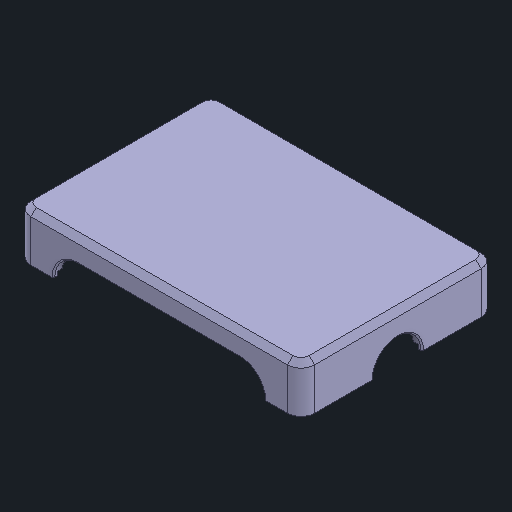
# Autodesk Inventor part: case2
Saved by Autodesk Inventor 2026.2 (Build 302298000, 298)
## iProperties
Created: 2025-10-05
Part Number: case2
Material: Generic
Document SubType Name: Modeling
Designer: micyg
Density: 1 g/cm^3
Appearance: Default
Sheet Metal Rule: Default
Author: micyg
## iProperties of the stored document case2_3DPrint.ipt
Created: 2025-10-05
Part Number: case2_3DPrint
Material: Generic
Document SubType Name: Modeling
Designer: micyg
Density: 1 g/cm^3
Appearance: Default
Author: micyg
Autodesk Inventor part; units mm, degrees
ref_plane "YZ Plane" through (0, 0, 0) normal (1, 0, 0) x (0, 1, 0)
ref_plane "XZ Plane" through (0, 0, 0) normal (0, 1, 0) x (-1, 0, 0)
ref_plane "XY Plane" through (0, 0, 0) normal (0, 0, 1) x (1, 0, 0)
sketch "Sketch1" plane through (0, 0, 0) normal (0, 1, 0) x (-1, 0, 0)
  line L0 (0, 0) -> (104.9, 0)
  line L1 (104.9, 0) -> (104.9, -71.6)
  line L2 (104.9, -71.6) -> (0, -71.6)
  line L3 (0, -71.6) -> (0, 0)
  dimension "d0" = 104.9
  dimension "d1" = 71.6
  constraints: 8 end point, 2 parallel, 1 horizontal, 1 perpendicular
  measures "d0" distance of L1.end L2.end
  measures "d1" distance of L0.end L1.end
extrude "Extrusion1" add sketch "Sketch1" along normal blind 17.5
fillet "Fillet1" radius 5 4 edges at (-104.9, 8.75, 0) (0, 8.75, 0) (-104.9, 8.75, -71.6) (0, 8.75, -71.6)
chamfer "Chamfer1" distance 2 angle 45 8 edges at (-52.45, 17.5, 0) (-1.4645, 17.5, -1.4645) (0, 17.5, -35.8) (-1.4645, 17.5, -70.1355) (-52.45, 17.5, -71.6) (-103.4355, 17.5, -70.1355) (-104.9, 17.5, -35.8) (-103.4355, 17.5, -1.4645)
shell "Shell2" thickness 3 removed faces 1 at (-68.2667, 0, -47.7333)
ref_plane "Work Plane2" through (-52.45, 0, 0) normal (1, 0, 0) x (0, 1, 0)
ref_plane "Work Plane3" through (0, 0, -35.8) normal (0, 0, -1) x (-1, 0, 0)
ref_plane "Work Plane4" through (0, 1.915, 0) normal (0, -1, 0) x (1, 0, 0)
sketch "Sketch19" plane through (-52.45, 0, 0) normal (1, 0, 0) x (0, 1, 0)
  line L0 (0, -3) -> (14.2574, -3) projected
  line L1 (14.2574, -3) -> (0, -3) projected
  line L2 (14.5, -5.7) -> (8.5, -5.7)
  line L3 (7.5, -5.7) -> (8.5, -6.7) construction
  line L4 (8.5, -6.7) -> (8.5, -5.7)
  line L5 (8.5, -5.7) -> (7.5, -5.7) construction
  line L6 (8.5, -6.7) -> (14.5, -12.7)
  line L7 (0, -66.6) -> (0, -71.6) projected
  line L8 (0, -5) -> (0, -66.6) projected
  line L9 (0, 0) -> (0, -5) projected
  line L10 (0, -5) -> (0, 0) projected
  line L11 (0, -66.6) -> (0, -5) projected
  line L12 (0, -71.6) -> (0, -66.6) projected
  line L13 (14.5, -3.2426) -> (14.5, -5) projected
  line L14 (14.5, -5) -> (14.5, -66.6) projected
  line L15 (14.5, -66.6) -> (14.5, -68.3574) projected
  line L16 (14.5, -68.3574) -> (14.5, -66.6) projected
  line L17 (14.5, -66.6) -> (14.5, -5) projected
  line L18 (14.5, -5) -> (14.5, -3.2426) projected
  dimension "d104" = 2.7
  dimension "d105" = 1
  dimension "d157" = 45
  dimension "d179" = 6
  constraints: 10 end point, 2 perpendicular, 2 point on line, 1 collinear
  measures "d104" distance between parallel lines of L0 L2
  measures "d105" distance from line of L3.end L2
  measures "d157" angle of L17 L6
  measures "d179" distance between parallel lines of L17 L4
extrude "Extrusion15" add sketch "Sketch19" against normal up to surface (49.45 mm away)
mirror "Mirror9" about plane through (-52.45, 0, 0) normal (1, 0, 0) of "Extrusion15"
mirror "Mirror10" about plane through (0, 0, -35.8) normal (0, 0, -1) of "Extrusion15", "Mirror9"
sketch "Sketch9" plane through (0, 1.915, 0) normal (0, -1, 0) x (1, 0, 0)
  arc A0 (-5, -71.6) -> (0, -66.6) centre (-5, -66.6) ccw projected
  line L0 (0, -5) -> (0, -66.6) projected
  arc A1 (0, -5) -> (-5, 0) centre (-5, -5) ccw projected
  line L1 (-99.9, 0) -> (-5, 0) projected
  arc A2 (-99.9, 0) -> (-104.9, -5) centre (-99.9, -5) ccw projected
  line L2 (-104.9, -66.6) -> (-104.9, -5) projected
  arc A3 (-104.9, -66.6) -> (-99.9, -71.6) centre (-99.9, -66.6) ccw projected
  line L3 (-5, -71.6) -> (-99.9, -71.6) projected
  line L4 (-96.4, -8.3) -> (-8.4, -8.3) construction
  line L5 (-8.4, -8.3) -> (-8.4, -63.3) construction
  line L6 (-8.4, -63.3) -> (-96.4, -63.3) construction
  line L7 (-96.4, -63.3) -> (-96.4, -8.3) construction
  circle A4 centre (-96.4, -8.3) radius 1.5
  circle A5 centre (-8.4, -8.3) radius 1.5
  circle A6 centre (-96.4, -63.3) radius 1.5
  circle A7 centre (-8.4, -63.3) radius 1.5
  line L8 (-52.4, -8.3) -> (-52.4, -63.3) construction
  line L9 (-101.4, -3.3) -> (-3.4, -3.3) construction
  line L10 (-3.4, -3.3) -> (-3.4, -68.3) construction
  line L11 (-3.4, -68.3) -> (-101.4, -68.3) construction
  line L12 (-101.4, -68.3) -> (-101.4, -3.3) construction
  line L13 (-101.4, -35.8) -> (-3.4, -35.8) construction
  line L14 (-52.45, 0) -> (-52.45, -71.6) construction
  line L15 (-104.9, -35.8) -> (0, -35.8) construction
  line L16 (-92.9, -3) -> (-92.9, -8.3)
  line L17 (-102.2, -11.8) -> (-102.2, -5)
  arc A8 (-96.4, -11.8) -> (-92.9, -8.3) centre (-96.4, -8.3) ccw
  line L18 (-96.4, -11.8) -> (-102.2, -11.8)
  line L19 (-100.2, -3) -> (-92.9, -3)
  line L20 (-92.9, -68.6) -> (-92.9, -63.3)
  arc A9 (-92.9, -63.3) -> (-96.4, -59.8) centre (-96.4, -63.3) ccw
  line L21 (-96.4, -59.8) -> (-102.2, -59.8)
  arc A10 (-11.9, -8.3) -> (-8.4, -11.8) centre (-8.4, -8.3) ccw
  line L22 (-3, -11.8) -> (-3, -5)
  line L23 (-11.9, -3) -> (-11.9, -8.3)
  line L24 (-8.4, -11.8) -> (-3, -11.8)
  line L25 (-5, -3) -> (-11.9, -3)
  arc A11 (-8.4, -59.8) -> (-11.9, -63.3) centre (-8.4, -63.3) ccw
  line L26 (-11.9, -68.6) -> (-11.9, -63.3)
  line L27 (-8.4, -59.8) -> (-3, -59.8)
  line L28 (-92.9, -3) -> (-94.9, -3)
  line L29 (-94.9, -3) -> (-94.9, -5.7)
  line L30 (-94.9, -5.7) -> (-92.9, -5.7)
  line L31 (-92.9, -5.7) -> (-92.9, -3)
  line L32 (-11.9, -3) -> (-9.9, -3)
  line L33 (-9.9, -3) -> (-9.9, -5.7)
  line L34 (-9.9, -5.7) -> (-11.9, -5.7)
  line L35 (-11.9, -5.7) -> (-11.9, -3)
  line L36 (-94.9, -68.6) -> (-94.9, -65.9)
  line L37 (-94.9, -65.9) -> (-92.9, -65.9)
  line L38 (-9.9, -68.6) -> (-9.9, -65.9)
  line L39 (-9.9, -65.9) -> (-11.9, -65.9)
  arc A12 (-3, -5) -> (-5, -3) centre (-5, -5) ccw projected
  line L40 (-5, -3) -> (-99.9, -3) projected
  line L41 (-3, -66.6) -> (-3, -5) projected
  arc A13 (0, -5) -> (-5, 0) centre (-5, -5) ccw projected
  line L42 (0, -5) -> (0, -66.6) projected
  line L43 (-99.9, 0) -> (-5, 0) projected
  arc A14 (-3, -5) -> (-5, -3) centre (-5, -5) ccw projected
  line L44 (-5, -3) -> (-99.9, -3) projected
  line L45 (-3, -66.6) -> (-3, -5) projected
  arc A15 (0, -5) -> (-5, 0) centre (-5, -5) ccw projected
  line L46 (0, -5) -> (0, -66.6) projected
  line L47 (-99.9, 0) -> (-5, 0) projected
  arc A16 (-5, -68.6) -> (-3, -66.6) centre (-5, -66.6) ccw projected
  line L48 (-5, -68.6) -> (-99.9, -68.6) projected
  arc A17 (-101.9, -66.6) -> (-99.9, -68.6) centre (-99.9, -66.6) ccw projected
  line L49 (-101.9, -66.6) -> (-101.9, -5) projected
  arc A18 (-99.9, -3) -> (-101.9, -5) centre (-99.9, -5) ccw projected
  line L50 (-99.9, -3) -> (-5, -3) projected
  arc A19 (-3, -5) -> (-5, -3) centre (-5, -5) ccw projected
  line L51 (-3, -5) -> (-3, -66.6) projected
  arc A20 (-5, -71.6) -> (0, -66.6) centre (-5, -66.6) ccw projected
  line L52 (0, -5) -> (0, -66.6) projected
  arc A21 (0, -5) -> (-5, 0) centre (-5, -5) ccw projected
  line L53 (-99.9, 0) -> (-5, 0) projected
  arc A22 (-99.9, 0) -> (-104.9, -5) centre (-99.9, -5) ccw projected
  line L54 (-104.9, -66.6) -> (-104.9, -5) projected
  arc A23 (-104.9, -66.6) -> (-99.9, -71.6) centre (-99.9, -66.6) ccw projected
  line L55 (-5, -71.6) -> (-99.9, -71.6) projected
  line L56 (-101.9, -6.7) -> (-101.9, -5.7) projected
  line L57 (-3, -6.7) -> (-101.9, -6.7) construction
  line L58 (-3, -5.7) -> (-3, -6.7) projected
  line L59 (-101.9, -5.7) -> (-3, -5.7) construction
  line L60 (-101.9, -65.9) -> (-101.9, -64.9) projected
  line L61 (-3, -65.9) -> (-101.9, -65.9) construction
  line L62 (-3, -64.9) -> (-3, -65.9) projected
  line L63 (-101.9, -64.9) -> (-3, -64.9) construction
  arc A24 (-5, -68.6) -> (-3, -66.6) centre (-5, -66.6) ccw projected
  arc A25 (-99.9, -3) -> (-101.9, -5) centre (-99.9, -5) ccw projected
  line L64 (-101.9, -5) -> (-101.9, -66.6) projected
  arc A26 (-101.9, -66.6) -> (-99.9, -68.6) centre (-99.9, -66.6) ccw projected
  line L65 (-99.9, -68.6) -> (-5, -68.6) projected
  arc A27 (-5, -71.6) -> (0, -66.6) centre (-5, -66.6) ccw projected
  line L66 (-5, -71.6) -> (-99.9, -71.6) projected
  arc A28 (-104.9, -66.6) -> (-99.9, -71.6) centre (-99.9, -66.6) ccw projected
  line L67 (-104.9, -66.6) -> (-104.9, -5) projected
  arc A29 (-99.9, 0) -> (-104.9, -5) centre (-99.9, -5) ccw projected
  arc A30 (-5, -68.6) -> (-3, -66.6) centre (-5, -66.6) ccw projected
  arc A31 (-99.9, -3) -> (-101.9, -5) centre (-99.9, -5) ccw projected
  line L68 (-101.9, -5) -> (-101.9, -66.6) projected
  arc A32 (-101.9, -66.6) -> (-99.9, -68.6) centre (-99.9, -66.6) ccw projected
  line L69 (-99.9, -68.6) -> (-5, -68.6) projected
  arc A33 (-5, -71.6) -> (0, -66.6) centre (-5, -66.6) ccw projected
  line L70 (-5, -71.6) -> (-99.9, -71.6) projected
  arc A34 (-104.9, -66.6) -> (-99.9, -71.6) centre (-99.9, -66.6) ccw projected
  line L71 (-104.9, -66.6) -> (-104.9, -5) projected
  arc A35 (-99.9, 0) -> (-104.9, -5) centre (-99.9, -5) ccw projected
  point P0 (-52.4, -35.8)
  point P1 (-11.9, -5.7)
  point P2 (-11.9, -65.9)
  point P3 (-92.9, -65.9)
  point P4 (-9.9, -3)
  point P5 (-101.9, -59.8)
  point P6 (-94.9, -68.6)
  point P7 (-101.9, -11.8)
  point P8 (-9.9, -68.6)
  dimension "d137" = 88
  dimension "d138" = 55
  dimension "d139" = 3
  dimension "d140" = 3
  dimension "d141" = 3
  dimension "d142" = 3
  dimension "d143" = 98
  dimension "d144" = 65
  dimension "d147" = 2
  dimension "d148" = 2
  dimension "d150" = 2
  dimension "d192" = 0.5
  constraints: 70 end point, 16 symmetric about line, 11 parallel, 10 midpoint, 8 centre point, 8 point on circle, 7 horizontal, 6 perpendicular, 5 coincident, 5 point on line, 4 tangent, 1 collinear, 6 other
  measures "d137" distance of L4.start L4.end
  measures "d138" distance of L6.end L4.start
  measures "d139" diameter of A4
  measures "d140" diameter of A7
  measures "d141" diameter of A5
  measures "d142" diameter of A6
  measures "d143" distance of L9.start L9.end
  measures "d144" distance of L12.start L9.start
  measures "d147" radial gap between concentric circles of A4 A8
  measures "d148" radial gap between concentric circles of A10 A5
  measures "d150" distance between parallel lines of L16 L29
  measures "d192" distance between parallel lines of L49 L12
extrude "Extrusion13" add sketch "Sketch9" against normal up to surface (12.585 mm away) contours L16 A8 L18 L49 A18 L19 L29 L30 | L34 L33 L25 A12 L22 L24 A10 L23 | L21 A9 L20 L37 L36 L48 A17 L49 | L41 A16 L48 L38 L39 L26 A11 L27
ref_plane "Work Plane6" through (0, 0, -23.8) normal (0, 0, -1) x (-1, 0, 0)
sketch "Sketch22" plane through (0, 0, -23.8) normal (0, 0, -1) x (-1, 0, 0)
  line L0 (3, 2.5) -> (15, 14.5)
  line L1 (89.9, 14.5) -> (102.05, 2.35)
  line L2 (3, 1.915) -> (3, 13.6) projected
  line L3 (3, 1.915) -> (3, 0) projected
  line L4 (3, 0) -> (3, 1.915) projected
  line L5 (3.2426, 14.5) -> (101.6574, 14.5) projected
  line L6 (101.6574, 14.5) -> (3.2426, 14.5) projected
  line L7 (101.9, 14.2574) -> (101.6574, 14.5) projected
  line L8 (101.6574, 14.5) -> (101.9, 14.2574) projected
  line L9 (101.9, 1.915) -> (101.9, 0) projected
  line L10 (101.9, 0) -> (101.9, 1.915) projected
  line L11 (52.45, -3.5) -> (52.45, 21) projected
  line L12 (101.9, 13.6) -> (101.9, 14.2574) projected
  line L13 (101.9, 14.2574) -> (101.9, 13.6) projected
  line L14 (3.2426, 14.5) -> (3, 14.2574) projected
  line L15 (3, 14.2574) -> (3.2426, 14.5) projected
  line L16 (3, 13.6) -> (3, 14.2574) projected
  line L17 (3, 14.2574) -> (3, 13.6) projected
  line L18 (9.9, 14.5) -> (94.9, 14.5) projected
  line L19 (94.9, 14.5) -> (9.9, 14.5) projected
  line L20 (9.9, 14.5) -> (94.9, 14.5) projected
  line L21 (94.9, 14.5) -> (9.9, 14.5) projected
  line L22 (101.9, 1.915) -> (101.9, 13.6) projected
  line L23 (101.9, 13.6) -> (101.9, 1.915) projected
  line L24 (3, 13.6) -> (3, 1.915) projected
  point P0 (89.9, 14.5)
  point P1 (3, 14.2574)
  point P2 (3.2426, 14.5)
  dimension "d184" = 12
  dimension "d185" = 45
  constraints: 4 end point, 3 point on line, 1 other
  measures "d184" distance from line of L5 L0.start
  measures "d185" angle of L6 L0
extrude "Extrusion18" add sketch "Sketch22" along normal mid plane 2 contours L2 L16 L14 L5 L0
mirror "Mirror12" about plane through (0, 0, -35.8) normal (0, 0, -1) of "Extrusion18"
sketch "Sketch26" plane through (0, 1.915, 0) normal (0, -1, 0) x (1, 0, 0)
  line L0 (-3, -59.8) -> (-3, -11.8) projected
  line L1 (0, -5) -> (0, -66.6) projected
  arc A0 (-5, -71.6) -> (0, -66.6) centre (-5, -66.6) ccw projected
  line L2 (-5, -71.6) -> (-99.9, -71.6) projected
  line L3 (-9.9, -5.7) -> (-9.9, -3) projected
  arc A1 (-3, -5) -> (-5, -3) centre (-5, -5) ccw projected
  arc A2 (0, -5) -> (-5, 0) centre (-5, -5) ccw projected
  line L4 (-99.9, 0) -> (-5, 0) projected
  line L5 (-9.9, -3) -> (-94.9, -3) projected
  line L6 (-11.9, -5.7) -> (-9.9, -5.7) projected
  line L7 (-11.9, -8.3) -> (-11.9, -5.7) projected
  arc A3 (-11.9, -8.3) -> (-8.4, -11.8) centre (-8.4, -8.3) ccw projected
  line L8 (-3, -11.8) -> (-8.4, -11.8) projected
  arc A4 (-99.9, 0) -> (-104.9, -5) centre (-99.9, -5) ccw projected
  line L9 (-104.9, -66.6) -> (-104.9, -5) projected
  arc A5 (-104.9, -66.6) -> (-99.9, -71.6) centre (-99.9, -66.6) ccw projected
  circle A6 centre (-96.4, -63.3) radius 1.5 projected
  circle A7 centre (-96.4, -8.3) radius 1.5 projected
  circle A8 centre (-8.4, -8.3) radius 1.5 projected
  circle A9 centre (-8.4, -63.3) radius 1.5 projected
  circle A10 centre (-8.4, -8.3) radius 1.5 projected
  circle A11 centre (-96.4, -63.3) radius 1.5 projected
  circle A12 centre (-8.4, -63.3) radius 1.5 projected
  circle A13 centre (-96.4, -8.3) radius 1.5 projected
  line L10 (-92.9, -5.7) -> (-92.9, -8.3) projected
  arc A14 (-96.4, -11.8) -> (-92.9, -8.3) centre (-96.4, -8.3) ccw projected
  line L11 (-96.4, -11.8) -> (-101.9, -11.8) projected
  line L12 (-101.9, -11.8) -> (-101.9, -5) projected
  arc A15 (-99.9, -3) -> (-101.9, -5) centre (-99.9, -5) ccw projected
  line L13 (-99.9, -3) -> (-94.9, -3) projected
  line L14 (-94.9, -3) -> (-94.9, -5.7) projected
  line L15 (-94.9, -5.7) -> (-92.9, -5.7) projected
  line L16 (-101.9, -11.8) -> (-101.9, -59.8) projected
  line L17 (-101.9, -66.6) -> (-101.9, -59.8) projected
  arc A16 (-101.9, -66.6) -> (-99.9, -68.6) centre (-99.9, -66.6) ccw projected
  line L18 (-94.9, -68.6) -> (-99.9, -68.6) projected
  line L19 (-94.9, -65.9) -> (-94.9, -68.6) projected
  line L20 (-92.9, -65.9) -> (-94.9, -65.9) projected
  line L21 (-92.9, -63.3) -> (-92.9, -65.9) projected
  arc A17 (-92.9, -63.3) -> (-96.4, -59.8) centre (-96.4, -63.3) ccw projected
  line L22 (-101.9, -59.8) -> (-96.4, -59.8) projected
  line L23 (-8.4, -59.8) -> (-3, -59.8) projected
  arc A18 (-8.4, -59.8) -> (-11.9, -63.3) centre (-8.4, -63.3) ccw projected
  line L24 (-11.9, -65.9) -> (-11.9, -63.3) projected
  line L25 (-9.9, -65.9) -> (-11.9, -65.9) projected
  line L26 (-9.9, -68.6) -> (-9.9, -65.9) projected
  line L27 (-94.9, -68.6) -> (-9.9, -68.6) projected
  line L28 (-9.9, -3) -> (-5, -3) projected
  line L29 (-3, -11.8) -> (-3, -5) projected
  line L30 (-3, -66.6) -> (-3, -59.8) projected
  arc A19 (-5, -68.6) -> (-3, -66.6) centre (-5, -66.6) ccw projected
  line L31 (-5, -68.6) -> (-9.9, -68.6) projected
  point P0 (0, 0)
extrude "Extrusion21" cut sketch "Sketch26" against normal up to surface (12.585 mm away) contours A6 | A7 | A8 | A9
sketch "Sketch30" plane through (0, 0, -5) normal (1, 0, 0) x (0, 0, -1)
  line L0 (0, 15.5) -> (61.6, 15.5) construction
  line L1 (0, 0) -> (0, 15.5) construction
  line L2 (0, 0) -> (61.6, 0) construction
  line L3 (61.6, 15.5) -> (61.6, 0) construction
  line L4 (30.8, 22.8) -> (30.8, -14.3) construction
  circle A0 centre (30.8, 0) radius 9
  point P0 (-5, 0)
  dimension "d160" = 18
  constraints: 1 centre point, 1 midpoint, 1 point on line
  measures "d160" diameter of A0
extrude "Extrusion22" cut sketch "Sketch30" against normal up to surface (3 mm away)
sketch "Sketch31" plane through (-5, 0, -71.6) normal (0, 0, -1) x (-1, 0, 0)
  line L0 (17.55, -9) -> (47.6, -9)
  arc A0 (17.55, 9) -> (17.55, -9) centre (17.55, 0) ccw
  line L1 (54.189, 9) -> (17.55, 9)
  line L2 (77.55, -9) -> (47.6, -9)
  arc A1 (77.55, -9) -> (77.55, 9) centre (77.55, 0) ccw
  line L3 (54.189, 9) -> (77.55, 9)
  line L4 (86.55, 9) -> (8.55, 9) construction
  line L5 (8.55, 9) -> (8.55, -9) construction
  line L6 (8.55, -9) -> (86.55, -9) construction
  line L7 (86.55, -9) -> (86.55, 9) construction
  line L8 (86.55, 9) -> (8.55, -9) construction
  line L9 (8.55, 9) -> (86.55, -9) construction
  line L10 (0, 15.5) -> (94.9, 15.5) projected
  line L11 (0, 0) -> (0, 15.5) projected
  line L12 (0, 0) -> (94.9, 0) projected
  line L13 (94.9, 15.5) -> (94.9, 0) projected
  line L14 (47.45, -14.3) -> (47.45, 22.8) projected
  point P0 (47.55, 0)
  point P1 (47.55, 0)
  point P2 (47.55, 0)
  dimension "d163" = 9
  dimension "d164" = 78
  dimension "d168" = 0.1
  constraints: 20 end point, 6 tangent, 4 midpoint, 4 point on circle, 3 collinear, 3 parallel, 3 point on line, 2 centre point, 1 horizontal, 1 perpendicular, 1 other
  measures "d163" radius of A0
  measures "d164" distance between parallel lines of L5 L7
extrude "Extrusion23" cut sketch "Sketch31" against normal up to surface (3 mm away) contours A0 L12 L14 L0 | L14 L12 A1 L2 L0 | A0 L1 L14 L12 | L14 L1 L3 A1 L12
mirror "Mirror13" about plane through (0, 0, -35.8) normal (0, 0, -1) of "Extrusion23"
sketch "Sketch33" plane through (0, 0, 0) normal (0, -1, 0) x (1, 0, 0)
  line L0 (-91.55, -3) -> (-91.55, 0) projected
  line L1 (-99.9, 0) -> (-91.55, 0) projected
  arc A0 (-99.9, 0) -> (-104.9, -5) centre (-99.9, -5) ccw projected
  line L2 (-104.9, -66.6) -> (-104.9, -5) projected
  arc A1 (-104.9, -66.6) -> (-99.9, -71.6) centre (-99.9, -66.6) ccw projected
  line L3 (-91.55, -71.6) -> (-99.9, -71.6) projected
  line L4 (-91.55, -71.6) -> (-91.55, -68.6) projected
  line L5 (-91.55, -68.6) -> (-99.9, -68.6) projected
  arc A2 (-101.9, -66.6) -> (-99.9, -68.6) centre (-99.9, -66.6) ccw projected
  line L6 (-101.9, -66.6) -> (-101.9, -5) projected
  arc A3 (-99.9, -3) -> (-101.9, -5) centre (-99.9, -5) ccw projected
  line L7 (-99.9, -3) -> (-91.55, -3) projected
  line L8 (-13.55, 0) -> (-13.55, -3) projected
  line L9 (-13.55, -3) -> (-5, -3) projected
  arc A4 (-3, -5) -> (-5, -3) centre (-5, -5) ccw projected
  line L10 (-3, -5) -> (-3, -26.8) projected
  line L11 (-3, -26.8) -> (0, -26.8) projected
  line L12 (0, -5) -> (0, -26.8) projected
  arc A5 (0, -5) -> (-5, 0) centre (-5, -5) ccw projected
  line L13 (-13.55, 0) -> (-5, 0) projected
  line L14 (-13.55, -68.6) -> (-13.55, -71.6) projected
  line L15 (-5, -71.6) -> (-13.55, -71.6) projected
  arc A6 (-5, -71.6) -> (0, -66.6) centre (-5, -66.6) ccw projected
  line L16 (0, -44.8) -> (0, -66.6) projected
  line L17 (0, -44.8) -> (-3, -44.8) projected
  line L18 (-3, -44.8) -> (-3, -66.6) projected
  arc A7 (-5, -68.6) -> (-3, -66.6) centre (-5, -66.6) ccw projected
  line L19 (-5, -68.6) -> (-13.55, -68.6) projected
  arc A8 (-5, -70.2) -> (-1.4, -66.6) centre (-5, -66.6) ccw
  line L20 (-5, -70.2) -> (-13.55, -70.2)
  line L21 (-1.4, -44.8) -> (-1.4, -66.6)
  line L22 (-13.55, -1.4) -> (-5, -1.4)
  arc A9 (-1.4, -5) -> (-5, -1.4) centre (-5, -5) ccw
  line L23 (-1.4, -5) -> (-1.4, -26.8)
  line L24 (-103.5, -5) -> (-103.5, -66.6)
  arc A10 (-103.5, -66.6) -> (-99.9, -70.2) centre (-99.9, -66.6) ccw
  line L25 (-99.9, -70.2) -> (-91.55, -70.2)
  line L26 (-91.55, -1.4) -> (-99.9, -1.4)
  arc A11 (-99.9, -1.4) -> (-103.5, -5) centre (-99.9, -5) ccw
  line L27 (-13.55, 0) -> (-13.55, -3) projected
  line L28 (-91.55, -71.6) -> (-91.55, -68.6) projected
  line L29 (-91.55, -3) -> (-91.55, 0) projected
  line L30 (-3, -44.8) -> (-3, -26.8) projected
  line L31 (-1.4, -44.8) -> (-3, -44.8)
  line L32 (-3, -44.8) -> (-3, -26.8)
  line L33 (-3, -26.8) -> (-1.4, -26.8)
  line L34 (-1.4, -26.8) -> (-1.4, -44.8)
  line L35 (-91.55, -1.4) -> (-13.55, -1.4)
  line L36 (-13.55, -1.4) -> (-13.55, -3)
  line L37 (-13.55, -3) -> (-91.55, -3)
  line L38 (-91.55, -3) -> (-91.55, -1.4)
  line L39 (-5, -68.6) -> (-13.55, -68.6) projected
  line L40 (-13.55, -68.6) -> (-91.55, -68.6)
  line L41 (-91.55, -68.6) -> (-91.55, -70.2)
  line L42 (-91.55, -70.2) -> (-13.55, -70.2)
  line L43 (-13.55, -70.2) -> (-13.55, -68.6)
  point P0 (0, 0)
  point P1 (-13.55, -70.2)
  dimension "d174" = 1.4
  dimension "d175" = 1.4
  dimension "d176" = 1.4
  constraints: 38 end point, 8 point on circle, 6 parallel, 6 point on line, 4 centre point, 3 horizontal, 3 perpendicular, 2 tangent, 6 other
  measures "d174" distance between parallel lines of L1 L26
  measures "d175" distance between parallel lines of L13 L22
  measures "d176" distance between parallel lines of L16 L21
extrude "Extrusion25" cut sketch "Sketch33" against normal blind 1.6 contours L7 A3 L6 A2 L5 L4 L25 A10 L24 A11 L26 L0 | L0 L35 L8 L37 | L8 L22 A9 L23 L11 L10 A4 L9 | L11 L34 L17 L30 | L40 L14 L42 L4 | L17 L21 A8 L20 L14 L19 A7 L18
sketch "Sketch34" plane through (0, 0, -24.8) normal (0, 0, -1) x (-1, 0, 0)
  line L0 (3, 14.2574) -> (3, 2.5) projected
  line L1 (3.2426, 14.5) -> (3, 14.2574) projected
  line L2 (15, 14.5) -> (3.2426, 14.5) projected
  line L3 (15, 14.5) -> (3, 2.5) construction
  line L4 (15, 14.5) -> (3.2426, 14.5) projected
  line L5 (3.2426, 14.5) -> (15, 14.5) projected
  line L6 (101.6574, 14.5) -> (3.2426, 14.5) projected
  line L7 (3.2426, 14.5) -> (15, 14.5) projected
  line L8 (15, 14.5) -> (3.2426, 14.5) projected
  line L9 (3.2426, 14.5) -> (101.6574, 14.5) projected
  line L10 (5.6, 14.5) -> (5.6, 8.5)
  line L11 (5.6, 7.5) -> (6.6, 8.5) construction
  line L12 (5.6, 8.5) -> (6.6, 8.5)
  line L13 (6.6, 8.5) -> (12.6, 14.5)
  line L14 (5.6, 8.5) -> (5.6, 7.5) construction
  line L15 (92.9, 8.5) -> (11.9, 8.5) projected
  line L16 (11.9, 8.5) -> (92.9, 8.5) projected
  point P0 (0, 0)
  point P1 (12.6, 14.5)
  dimension "d180" = 1
  dimension "d181" = 45
  dimension "d183" = 2.6
  constraints: 10 end point, 2 collinear, 2 point on line, 2 vertical, 1 horizontal
  measures "d180" distance from line of L11.end L10
  measures "d181" angle of L9 L13
  measures "d183" distance between parallel lines of L0 L10
extrude "Extrusion26" add sketch "Sketch34" along normal up to surface (22 mm away)
chamfer "Chamfer2" distance 0.5 angle 45 7 edges at (-16.186, 6.364, 0) (-52.55, 9, 0) (-88.914, 6.364, 0) (-16.186, 6.364, -71.6) (-52.55, 9, -71.6) (-88.914, 6.364, -71.6) (0, 9, -35.8)
equation "\"BendRadius\" = Thickness"
equation "\"BendReliefWidth\" = Thickness"
equation "\"BendReliefDepth\" = 0.5 * Thickness"
equation "\"CornerReliefSize\" = 4 * Thickness"
equation "\"MinimumRemnant\" = 2 * Thickness"
equation "\"TransitionRadius\" = BendRadius"
equation "\"JacobiRadiusSize\" = BendRadius"
equation "\"GapSize\" = Thickness"
equation "\"Thickness\" = 3.048"
body "Solid1"
